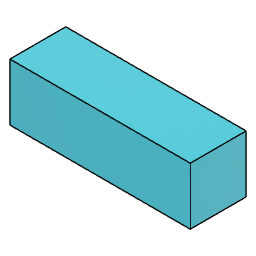
chassis_design_v1 (Autodesk Fusion 360 archive; units mm, degrees)
design "battery_placeholder"
Autodesk Fusion 360 part; units mm, degrees
sketch "Sketch1" plane through (0, 0, 0) normal (0, 1, 0) x (1, 0, 0)
  line L0 (0, 0) -> (-142, 0)
  line L1 (-142, 0) -> (-142, 44)
  line L2 (-142, 44) -> (0, 44)
  line L3 (0, 44) -> (0, 0)
  dimension "d4" = 142
  dimension "d5" = 44
  constraint horizontal L0
  constraint vertical L1
  constraint horizontal L2
  constraint vertical L3
  constraint coincident L0.start L3.end
  measures "d4" distance of L0.start L0.end
  measures "d5" distance of L0.start L2.end
extrude "Extrude1" add sketch "Sketch1" along normal blind 45
equation "length = 142 mm"
equation "width = 44 mm"
equation "height = 45 mm"
equation "d4 = length"
equation "d5 = width"
equation "d6 = height"

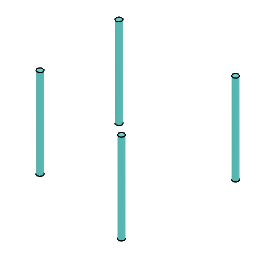
design "holes_for_lidar"
Autodesk Fusion 360 part; units mm, degrees
sketch "Sketch1" plane through (0, -46.9838, 0) normal (0, -1, 0) x (1, 0, 0)
  circle A0 centre (-44, 28.5052) radius 1.8916
  circle A1 centre (24.5, -33.5582) radius 1.8916
  circle A2 centre (-47, -27.1805) radius 1.8916
  circle A3 centre (20.5, 38.6499) radius 1.8916
  line L0 (-43.3254, -23.9949) -> (-40.6905, 25.4827)
  line L1 (-40.6905, 25.4827) -> (17.2228, 34.5914)
  line L2 (17.2228, 34.5914) -> (20.8403, -29.7179)
  line L3 (20.8403, -29.7179) -> (-43.3254, -23.9949)
  arc A4 (23.4796, -36.9062) -> (27.9945, -33.3616) centre (24.5, -33.5582) ccw
  line L4 (27.9945, -33.3616) -> (23.9696, 38.1893)
  arc A5 (23.9696, 38.1893) -> (19.9562, 42.1074) centre (20.5, 38.6499) ccw
  line L5 (19.9562, 42.1074) -> (-44.5438, 31.9627)
  arc A6 (-44.5438, 31.9627) -> (-47.495, 28.6914) centre (-44, 28.5052) ccw
  line L6 (-47.495, 28.6914) -> (-50.4346, -26.5069)
  arc A7 (-50.4346, -26.5069) -> (-47.3073, -30.667) centre (-47, -27.1805) ccw
  line L7 (-47.3073, -30.667) -> (23.4796, -36.9062)
  circle A8 centre (-44, 28.5052) radius 1.8916
  circle A9 centre (-47, -27.1805) radius 1.8916
  circle A10 centre (24.5, -33.5582) radius 1.8915
  circle A11 centre (20.5, 38.6499) radius 1.8915
  constraint concentric A0 A8
  constraint concentric A2 A9
  constraint concentric A1 A10
  constraint concentric A3 A11
extrude "Extrude1" add sketch "Sketch1" along normal blind 60 contours A0 A8 | A1 A10 | A2 A9 | A3 A11 makes body 1 at (18.8388, -86.9838, 37.7452) makes body 2 at (-46.7648, -86.9838, -25.3036) makes body 3 at (-43.7648, -86.9838, 30.3821) makes body 4 at (22.6178, -86.9838, -33.7465)

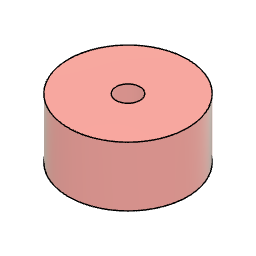
design "wheel placeholder"
Autodesk Fusion 360 part; units mm, degrees
sketch "Sketch1" plane through (0, 0, 0) normal (0, 1, 0) x (1, 0, 0)
  circle A0 centre (0, 0) radius 50
  circle A1 centre (0, 0) radius 10
  dimension "d1" = 100
  constraint coincident A0.centre A1.centre
  constraint concentric A0 A1
  measures "d1" diameter of A0
extrude "Extrude1" add sketch "Sketch1" along normal blind 50
equation "d1 = wheel_radius"
equation "d2 = wheel_height"
equation "wheel_height = 50 mm"
equation "wheel_radius = 100 mm"
